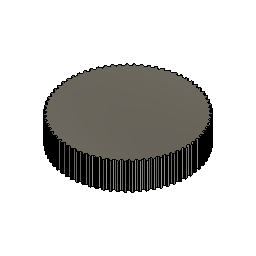
gear_71z (Autodesk Fusion 360 design; units mm, degrees)
Autodesk Fusion 360 part; units mm, degrees
sketch "Sketch1" plane through (0, 0, 0) normal (0, 0, 1) x (1, 0, 0) in component "gt2 pulley"
  circle A0 centre (0, 0) radius 22.6 construction
  circle A1 centre (0, 0) radius 21.596 construction
  line L0 (0, 0) -> (0, 22.6) construction
  line L1 (0, 0) -> (0.9997, 22.5779) construction
  line L2 (0, 0) -> (1.4054, 22.5563) construction
  circle A2 centre (0, 0) radius 22.346 construction
  arc A3 (0.3941, 22.2088) -> (0.4687, 21.913) centre (1.3896, 22.3028) ccw
  circle A4 centre (0, 0) radius 22.196 construction
  arc A5 (0.2463, 22.3446) -> (0, 22.346) centre (0, 0) ccw
  arc A6 (0.3941, 22.2088) -> (0.2463, 22.3446) centre (0.2447, 22.1947) ccw
  arc A7 (0.4687, 21.913) -> (0.9553, 21.5749) centre (0.9798, 22.1293) ccw
  arc A8 (0, 22.346) -> (-0.2463, 22.3446) centre (0, 0) ccw
  arc A9 (-0.2463, 22.3446) -> (-0.3941, 22.2088) centre (-0.2447, 22.1947) ccw
  arc A10 (-0.4687, 21.913) -> (-0.3941, 22.2088) centre (-1.3896, 22.3028) ccw
  arc A11 (-0.9554, 21.5749) -> (-0.4687, 21.913) centre (-0.9798, 22.1293) ccw
  arc A12 (0.9553, 21.5749) -> (-0.9553, 21.5749) centre (0, 0) ccw
  point P0 (1.3896, 22.3028)
  point P1 (0, 22.346)
  dimension "d18" = 45.2
  dimension "d19" = 2.535
  dimension "d22" = 1.004
  dimension "d24" = 0.75
  dimension "d26" = 1
  dimension "d27" = 0.15
  dimension "d28" = 0.15
  dimension "d47" = 0.555
  dimension "d52" = 3.812
  constraint coincident A0.centre A1.centre
  constraint coincident A0 L0.end
  constraint vertical L0
  constraint coincident A0 L1.end
  constraint coincident A0 L2.end
  constraint concentric A1 A2
  constraint coincident A1 A7.end
  constraint coincident L1 A7.end
  constraint coincident A2 P0
  constraint coincident L2 P0
  constraint coincident P0 A3.centre
  constraint coincident A2 P1
  constraint coincident L0 P1
  constraint concentric A2 A4
  constraint coincident P1 A5.end
  constraint coincident A4 A6.centre
  constraint coincident A3.start A6.start
  constraint tangent A3 A6
  constraint tangent A3 A7
  constraint symmetric L0 A7.end A12.end
  constraint symmetric L0 A3.start A9.end
  constraint symmetric L0 A3.end A10.start
  constraint symmetric L0 A3 A10
  constraint symmetric L0 A5.start A8.end
  constraint symmetric L0 P1 A5.end
  constraint symmetric L0 A5 A8
  constraint symmetric L0 A6 A9
  constraint symmetric L0 A7 A11
  constraint coincident A1 A11.start
  constraint tangent A1 A7
  constraint coincident L1 A7.centre
  measures "d18" diameter of A0
  measures "d19" angle of L0 L1
  measures "d22" distance of A0 A1
  measures "d24" distance of A1 A2
  measures "d26" radius of A3
  measures "d27" distance of A2 A4
  measures "d28" radius of A6
  measures "d47" radius of A7
extrude "Extrude1" add sketch "Sketch1" along normal blind 10 makes body 1
pattern_circular "C-Pattern1" count 71 over 360 about axis through (0, 0, 1.75) along (0, 0, 1) of bodies 1 makes body 2 at (-1.1674, 21.5644, 3.3333) makes body 3 at (-4.5317, 21.1152, 6.6667) makes body 4 at (-5.7688, 20.8113, 6.6667) makes body 5 at (-6.7845, 20.5026, 3.3333) makes body 6 at (-9.3429, 19.4704, 6.6667) makes body 7 at (-10.2884, 18.9878, 3.3333) makes body 8 at (-13.1364, 17.1413, 6.6667) makes body 9 at (-13.9629, 16.475, 6.6667) makes body 10 at (-15.5128, 15.0247, 6.6667) makes body 11 at (-16.78, 13.5949, 6.6667) makes body 12 at (-17.4278, 12.7539, 3.3333) makes body 13 at (-18.4867, 11.1637, 3.3333) makes body 14 at (-19.7591, 8.7159, 6.6667) makes body 15 at (-20.1635, 7.7343, 3.3333) makes body 16 at (-20.7682, 5.922, 3.3333) makes body 17 at (-21.2103, 4.0634, 3.3333) makes body 18 at (-21.5552, 1.3263, 6.6667) makes body 19 at (-21.5881, -0.584, 6.6667) makes body 20 at (-21.5333, -1.6441, 3.3333) makes body 21 at (-21.0098, -4.9977, 6.6667) makes body 22 at (-20.4859, -6.835, 6.6667) makes body 23 at (-20.3475, -7.2364, 6.6667) makes body 24 at (-19.6283, -9.0064, 3.3333) makes body 25 at (-18.32, -11.4352, 6.6667) makes body 26 at (-17.736, -12.3217, 3.3333) makes body 27 at (-16.5776, -13.8409, 3.3333) makes body 28 at (-15.2894, -15.2519, 3.3333) makes body 29 at (-13.8816, -16.5435, 3.3333) makes body 30 at (-11.6594, -18.1782, 6.6667) makes body 31 at (-10.1949, -19.0382, 6.6667) makes body 32 at (-8.4724, -19.8647, 6.6667) makes body 33 at (-5.8709, -20.7827, 6.6667) makes body 34 at (-5.4611, -20.8941, 3.3333) makes body 35 at (-3.5931, -21.295, 3.3333) makes body 36 at (-1.0613, -21.5699, 6.6667) makes body 37 at (0.2124, -21.595, 6.6667) makes body 38 at (2.7531, -21.4198, 6.6667) makes body 39 at (4.8426, -21.0461, 6.6667) makes body 40 at (5.871, -20.7827, 6.6667) makes body 41 at (8.8615, -19.6942, 6.6667) makes body 42 at (10.195, -19.0381, 6.6667) makes body 43 at (11.1182, -18.5141, 3.3333) makes body 44 at (13.3877, -16.9457, 6.6667) makes body 45 at (14.833, -15.6962, 6.6667) makes body 46 at (15.5864, -14.9483, 3.3333) makes body 47 at (16.8465, -13.5123, 3.3333) makes body 48 at (18.7556, -10.7058, 6.6667) makes body 49 at (18.9625, -10.335, 3.3333) makes body 50 at (20.1253, -7.8333, 6.6667) makes body 51 at (20.7388, -6.024, 6.6667) makes body 52 at (21.1901, -4.1675, 6.6667) makes body 53 at (21.4755, -2.2784, 6.6667) makes body 54 at (21.5615, -1.2203, 3.3333) makes body 55 at (21.585, 0.69, 3.3333) makes body 56 at (21.2103, 4.0635, 6.6667) makes body 57 at (21.1263, 4.4797, 3.3333) makes body 58 at (20.1635, 7.7345, 6.6667) makes body 59 at (20.0075, 8.1294, 3.3333) makes body 60 at (19.1128, 10.0543, 6.6667) makes body 61 at (17.4277, 12.754, 6.6667) makes body 62 at (17.1736, 13.0941, 3.3333) makes body 63 at (15.9491, 14.5607, 3.3333) makes body 64 at (14.1241, 16.337, 6.6667) makes body 65 at (13.1363, 17.1413, 3.3333) makes body 66 at (10.8439, 18.6761, 6.6667) makes body 67 at (9.1508, 19.5614, 6.6667) makes body 68 at (6.7844, 20.5027, 6.6667) makes body 69 at (5.5637, 20.867, 6.6667) makes body 70 at (3.6977, 21.2771, 6.6667) makes body 71 at (2.0143, 21.5019, 6.6667)
sketch "Sketch2" plane through (0, 0, 10) normal (0, 0, 1) x (-1, 0, 0)
  arc A0 (-14.7415, -16.6155) -> (-14.7176, -16.8148) centre (-14.6188, -16.7019) ccw
  arc A1 (-14.7176, -16.8148) -> (-14.3434, -17.1351) centre (0, 0) ccw
  arc A2 (-14.3434, -17.1351) -> (-14.1427, -17.128) centre (-14.247, -17.0201) ccw
  arc A3 (-13.8937, -16.9518) -> (-14.1427, -17.128) centre (-13.4475, -17.8468) ccw
  arc A4 (-13.3042, -17.0113) -> (-13.8937, -16.9518) centre (-13.6461, -17.4485) ccw
  arc A5 (-14.7556, -15.7689) -> (-13.3042, -17.0113) centre (0, 0) ccw
  arc A6 (-14.6059, -16.3422) -> (-14.7556, -15.7689) centre (-15.1348, -16.1742) ccw
  arc A7 (-14.7415, -16.6155) -> (-14.6059, -16.3422) centre (-15.5589, -16.0395) ccw
  circle A8 centre (0, 0) radius 21.596
  constraint concentric A1 A8
extrude "Extrude2" add sketch "Sketch2" against normal blind 10 contours A5 A8 bodies 1 2 3 4 5 6 7 8 9 10 11 12 13 14 15 16 17 18 19 20 21 22 23 24 25 26 27 28 29 30 31 32 33 34 35 36 37 38 39 40 41 42 43 44 45 46 47 48 49 50 51 52 53 54 55 56 57 58 59 60 61 62 63 64 65 66 67 68 69 70 71
extrude "Extrude4" [suppressed] in component "gt2 pulley"
pattern_circular "C-Pattern7" [suppressed] in component "gt2 pulley"
extrude "Extrude3" [suppressed] in component "gt2 pulley"
pattern_circular "C-Pattern6" [suppressed] in component "gt2 pulley"
extrude "Extrude2'" [suppressed] in component "gt2 pulley"
pattern_circular "C-Pattern5" [suppressed] in component "gt2 pulley"
extrude "Extrude1'" [suppressed] in component "gt2 pulley"
pattern_circular "C-Pattern4" [suppressed] in component "gt2 pulley"
pattern_circular "C-Pattern3" [suppressed] in component "gt2 pulley"
pattern_circular "C-Pattern2" [suppressed] in component "gt2 pulley"
pattern_circular "C-Pattern1'" [suppressed] in component "gt2 pulley"
copy_body "Body->Comp1" [suppressed] in component "Component"
copy_body "Body->Comp2" [suppressed] in component "Component'"
copy_body "Body->Comp3" [suppressed] in component "Component''"
copy_body "Body->Comp4" [suppressed] in component "Component'''"
copy_body "Body->Comp5" [suppressed] in component "Component''''"
copy_body "Body->Comp6" [suppressed] in component "Component'''''"
copy_body "Body->Comp7" [suppressed] in component "Component''''''"
copy_body "Body->Comp8" [suppressed] in component "Component'''''''"
copy_body "Body->Comp9" [suppressed] in component "Component''''''''"
copy_body "Body->Comp10" [suppressed] in component "Component'''''''''"
copy_body "Body->Comp11" [suppressed] in component "Component''''''''''"
copy_body "Body->Comp12" [suppressed] in component "Component'''''''''''"
copy_body "Body->Comp13" [suppressed] in component "Component''''''''''''"
copy_body "Body->Comp14" [suppressed] in component "Component'''''''''''''"
copy_body "Body->Comp15" [suppressed] in component "Component''''''''''''''"
copy_body "Body->Comp16" [suppressed] in component "Component'''''''''''''''"
copy_body "Body->Comp17" [suppressed] in component "Component''''''''''''''''"
copy_body "Body->Comp18" [suppressed] in component "Component'''''''''''''''''"
copy_body "Body->Comp19" [suppressed] in component "Component''''''''''''''''''"
copy_body "Body->Comp20" [suppressed] in component "Component'''''''''''''''''''"
component "gt2 pulley" placed x (1, 0, 0) y (0, 1, 0) z (0, 0, 1) at (0, 0, 0)
equation "NumTeeth = 71" comment "min 20"
equation "ToothPitch = 2 mm"
equation "PullyDia = NumTeeth * ToothPitch / PI"
equation "ToothAng = ( ( 360 / NumTeeth ) * 1 deg )"
equation "TransOffsetAngle = ToothAng * 0.2"
equation "Sholulder_Radius = 0.15 mm"
equation "Root_Radius = 0.555 mm"
equation "TransRadius = 1 mm"
equation "ToolHeight = 0.75 mm"
equation "PLD = 0.254 mm"
equation "d18 = PullyDia"
equation "d19 = ToothAng / 2"
equation "d22 = PLD + ToolHeight"
equation "d24 = ToolHeight"
equation "d26 = TransRadius"
equation "d27 = Sholulder_Radius"
equation "d31 = NumTeeth"
equation "d33 = NumTeeth"
equation "d35 = NumTeeth"
equation "d37 = NumTeeth"
equation "d41 = NumTeeth"
equation "d45 = NumTeeth"
equation "d47 = Root_Radius"
equation "d50 = NumTeeth"
